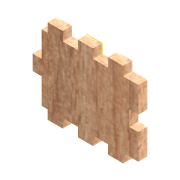
# Autodesk Inventor part: jotstick behuizing zijkant 2
Saved by Autodesk Inventor 2020.3 (Build 243373000, 373)
## iProperties
Created: 2020-12-09
Part Number: jotstick behuizing zijkant 2
Material: Wood (Birch)
Document SubType Name: Sheet Metal
Designer: Svend
Density: 0.55 g/cm^3
Sheet Metal Rule: Default_mm
Appearance: Birch - Natural Polished
Author: Svend
Autodesk Inventor part; units mm, degrees
ref_plane "YZ Plane" through (0, 0, 0) normal (1, 0, 0) x (0, 1, 0)
ref_plane "XZ Plane" through (0, 0, 0) normal (0, 1, 0) x (-1, 0, 0)
ref_plane "XY Plane" through (0, 0, 0) normal (0, 0, 1) x (1, 0, 0)
ref_plane "Work Plane1" through (20, 0, 0) normal (0, 0, 1) x (1, 0, 0)
sketch "Sketch1" plane through (20, 0, 0) normal (0, 0, 1) x (1, 0, 0)
  line L0 (-20, 0) -> (-10, 0) projected
  line L1 (-10, 0) -> (-10, 6) projected
  line L2 (-20, 6) -> (-10, 6) projected
  line L3 (-20, 0) -> (-20, 6) projected
  line L4 (0, 0) -> (10, 0) projected
  line L5 (10, 0) -> (10, 6) projected
  line L6 (0, 6) -> (10, 6) projected
  line L7 (0, 0) -> (0, 6) projected
  line L8 (20, 0) -> (30, 0) projected
  line L9 (30, 0) -> (30, 6) projected
  line L10 (20, 6) -> (30, 6) projected
  line L11 (20, 0) -> (20, 6) projected
  line L12 (-30, 0) -> (-24, 0) projected
  line L13 (-24, 0) -> (-24, 6) projected
  line L14 (-30, 6) -> (-24, 6) projected
  line L15 (-30, 0) -> (-30, 6) projected
  line L16 (-30, 0) -> (-20, 0) projected
  line L17 (-10, 0) -> (0, 0) projected
  line L18 (10, 0) -> (20, 0) projected
  line L19 (-24, -22) -> (40, -22) construction
  line L20 (-30, -24.5) -> (-30, -34.5) projected
  line L21 (-24, -24.5) -> (-30, -24.5) projected
  line L22 (-24, -34.5) -> (-24, -24.5) projected
  line L23 (-24, -34.5) -> (-30, -34.5) projected
  line L24 (34, -34.5) -> (40, -34.5) projected
  line L25 (40, -34.5) -> (40, -44) projected
  line L26 (34, -44) -> (40, -44) projected
  line L27 (34, -44) -> (34, -34.5) projected
  line L28 (34, -24.5) -> (40, -24.5) projected
  line L29 (34, -24.5) -> (34, -15) projected
  line L30 (34, -15) -> (40, -15) projected
  line L31 (40, -15) -> (40, -24.5) projected
  line L32 (-30, -24.5) -> (-30, -34.5) projected
  line L33 (-24, -24.5) -> (-30, -24.5) projected
  line L34 (-24, -34.5) -> (-24, -24.5) projected
  line L35 (-24, -34.5) -> (-30, -34.5) projected
  line L36 (-30, -24.5) -> (-30, -34.5) projected
  line L37 (-24, -24.5) -> (-30, -24.5) projected
  line L38 (-24, -34.5) -> (-24, -24.5) projected
  line L39 (-24, -34.5) -> (-30, -34.5) projected
  line L40 (40, -24.5) -> (40, -34.5) projected
  line L41 (34, -34.5) -> (40, -34.5) projected
  line L42 (34, -34.5) -> (34, -24.5) projected
  line L43 (34, -24.5) -> (40, -24.5) projected
  line L44 (-20, -44) -> (-10, -44) projected
  line L45 (-10, -44) -> (-10, -50) projected
  line L46 (-20, -50) -> (-10, -50) projected
  line L47 (-20, -44) -> (-20, -50) projected
  line L48 (0, -44) -> (10, -44) projected
  line L49 (10, -44) -> (10, -50) projected
  line L50 (0, -50) -> (10, -50) projected
  line L51 (0, -44) -> (0, -50) projected
  line L52 (20, -44) -> (30, -44) projected
  line L53 (30, -44) -> (30, -50) projected
  line L54 (20, -50) -> (30, -50) projected
  line L55 (20, -44) -> (20, -50) projected
  line L56 (-30, -44) -> (-20, -44) projected
  line L57 (-24, -34.5) -> (-24, -44) projected
  line L58 (30, -44) -> (40, -44) projected
  line L59 (-24, -44) -> (34, -44)
  line L60 (34, -44) -> (34, 0)
  line L61 (34, 0) -> (-24, 0)
  line L62 (-24, 0) -> (-24, -44)
  line L63 (-30, -15) -> (-30, -9) projected
  line L64 (-24, -9) -> (-30, -9) projected
  line L65 (-24, -9) -> (-24, -15) projected
  line L66 (-24, -15) -> (-30, -15) projected
  line L67 (-24, -9) -> (-30, -9)
  line L68 (-30, -9) -> (-30, 0)
  line L69 (-30, 0) -> (-24, 0)
  line L70 (-24, 0) -> (-24, -9)
  line L71 (-24, 0) -> (-20, 0)
  line L72 (-20, 0) -> (-20, 6)
  line L73 (-20, 6) -> (-24, 6)
  line L74 (-24, 6) -> (-24, 0)
  point P0 (-30, -29.5)
  point P1 (40, -32.6552)
  dimension "d4" = 44
  constraints: 26 end point, 11 symmetric about line, 6 parallel, 3 horizontal, 3 perpendicular
  measures "d4" distance of L60.end L59.end
extrude "Plate1" add sketch "Sketch1" along normal blind 6 contours L3 L2 L1 L0 | L16 L13 L73 L3 | L0 L17 L4 L18 L8 L61 L60 L29 L42 L27 L58 L52 L59 L48 L44 L56 L57 L22 L62 L16 | L62 L64 L68 L12 | L7 L6 L5 L4 | L62 L66 L63 L64 | L11 L10 L9 L8 | L22 L23 L20 L21 | L30 L31 L28 L29 | L44 L45 L46 L47 | L24 L25 L26 L27 | L48 L49 L50 L51 | L53 L54 L55 L52
equation "\"d3\" = Thickness"
equation "\"BendRadius\" = Thickness"
equation "\"BendReliefWidth\" = Thickness"
equation "\"BendReliefDepth\" = 0.5 * Thickness"
equation "\"CornerReliefSize\" = 4 * Thickness"
equation "\"MinimumRemnant\" = 2 * Thickness"
equation "\"TransitionRadius\" = BendRadius"
equation "\"JacobiRadiusSize\" = BendRadius"
equation "\"GapSize\" = Thickness"
equation "\"Thickness\" = 6"
body "Solid1"
